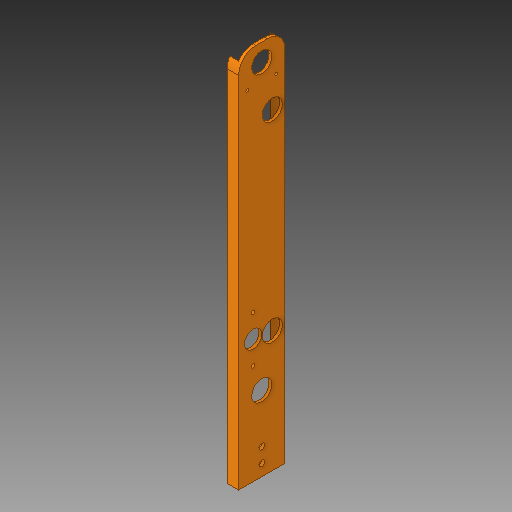
# Autodesk Inventor part: Front C Left
Saved by Autodesk Inventor 2017 (Build 210142000, 142)
## iProperties
Created: 2017-01-13
Part Number: Front C Left
Material: Generic
Document SubType Name: Modeling
Designer: Ben
Density: 1 g/cm^3
Appearance: Orange
Author: Ben
Autodesk Inventor part; units mm, degrees
ref_plane "YZ Plane" through (0, 0, 0) normal (1, 0, 0) x (0, 1, 0)
ref_plane "XZ Plane" through (0, 0, 0) normal (0, 1, 0) x (-1, 0, 0)
ref_plane "XY Plane" through (0, 0, 0) normal (0, 0, 1) x (1, 0, 0)
sketch "Sketch1" plane through (0, 0, 0) normal (1, 0, 0) x (0, 1, 0)
  line L0 (0, 0) -> (0, -50.8)
  line L1 (0, -50.8) -> (412.242, -50.8)
  line L2 (412.242, -50.8) -> (412.242, 0)
  line L3 (412.242, 0) -> (0, 0)
  line L4 (412.242, -25.4) -> (0, -25.4) construction
  circle A0 centre (82.042, -25.4) radius 11.1125
  circle A1 centre (393.192, -25.4) radius 11.1125
  line L5 (0, -13.97) -> (412.242, -13.97) construction
  line L6 (132.842, -13.97) -> (132.842, -36.83) construction
  line L7 (342.392, -13.97) -> (342.392, -36.83) construction
  circle A2 centre (132.842, -36.83) radius 11.1125
  circle A3 centre (342.392, -36.83) radius 11.1125
  line L8 (132.842, -36.83) -> (342.392, -36.83) construction
  line L9 (160.6042, -15.875) -> (109.8042, -15.875) construction
  circle A4 centre (135.2042, -15.875) radius 9.525
  circle A5 centre (160.6042, -15.875) radius 2.0193
  circle A6 centre (109.8042, -15.875) radius 2.0193
  circle A7 centre (374.142, -9.525) radius 1.5875 projected
  circle A8 centre (374.142, -41.275) radius 1.5875 projected
  circle A9 centre (12.7, -25.4) radius 3.175
  circle A10 centre (28.575, -25.4) radius 3.175
  dimension "d0" = 50.8
  dimension "d3" = 22.225
  dimension "d4" = 311.15
  dimension "d5" = 19.05
  dimension "d12" = 82.042
  dimension "d18" = 11.43
  dimension "d19" = 50.8
  dimension "d20" = 50.8
  dimension "d29" = 15.875
  dimension "d30" = 50.8
  dimension "d31" = 53.1622
  dimension "d35" = 4.0386
  dimension "d36" = 19.05
  dimension "d37" = 22.225
  dimension "d38" = 12.7
  dimension "d39" = 15.875
  dimension "d40" = 6.35
  constraints: 20 end point, 9 centre point, 8 point on line, 4 coincident, 4 equal radius, 3 midpoint, 3 parallel, 2 horizontal, 2 perpendicular, 2 vertical, 1 other
  measures "d0" distance of L0.start L0.end
  measures "d3" diameter of A0
  measures "d4" distance of A0.centre A1.centre
  measures "d5" distance from line of L2 A1.centre
  measures "d12" distance from line of L0 A0.centre
  measures "d18" distance between parallel lines of L5 L4
  measures "d19" horizontal distance of A0.centre L6.start
  measures "d20" horizontal distance of A1.centre L7.start
  measures "d29" distance between parallel lines of L3 L9
  measures "d30" distance of L9.start L9.end
  measures "d31" horizontal distance of A0.centre A4.centre
  measures "d35" diameter of A5
  measures "d36" diameter of A4
  measures "d37" diameter of A2
  measures "d38" distance from line of A9.centre L0
  measures "d39" distance of A9.centre A10.centre
  measures "d40" diameter of A9
extrude "Extrusion1" add sketch "Sketch1" along normal blind 3.175
sketch "Sketch2" plane through (0, 0, 0) normal (-1, 0, 0) x (0, 0, 1)
  line L0 (0, 412.242) -> (0, 0) projected
  line L1 (-50.8, 412.242) -> (0, 412.242) construction
  line L2 (0, 0) -> (-3.175, 0)
  line L3 (-3.175, 0) -> (-3.175, 412.242)
  line L4 (-3.175, 412.242) -> (0, 412.242)
  line L5 (0, 412.242) -> (0, 0)
  line L6 (-50.8, 0) -> (-50.8, 412.242) projected
  line L7 (-50.8, 0) -> (-47.625, 0)
  line L8 (-47.625, 0) -> (-47.625, 412.242)
  line L9 (-47.625, 412.242) -> (-50.8, 412.242)
  line L10 (-50.8, 412.242) -> (-50.8, 0)
  dimension "d13" = 3.175
  dimension "d14" = 3.175
  constraints: 16 end point, 4 parallel, 2 horizontal, 2 perpendicular, 2 point on line
  measures "d13" distance of L0.end L2.end
  measures "d14" distance of L6.start L7.end
extrude "Extrusion2" add sketch "Sketch2" along normal blind 9.525
fillet "Fillet2" radius 19.05 2 edges at (-3.175, 412.242, 0) (-3.175, 412.242, -50.8)
equation "\"d20\" = d19"
equation "\"d29\" = d23"
equation "\"d14\" = d13"
equation "\"d23\" = 15.875"
body "Solid1"
